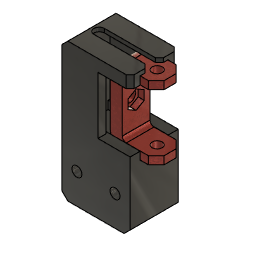
A Belt Tension Buddy_1x (Autodesk Fusion 360 design; units mm, degrees)
Autodesk Fusion 360 part; units mm, degrees
sketch "Sketch1" plane through (0, 0, 0) normal (0, 1, 0) x (1, 0, 0)
  line L0 (-15, 17.25) -> (15, 17.25)
  line L1 (15, 17.25) -> (15, -17.25)
  line L2 (15, -17.25) -> (-15, -17.25)
  line L3 (-15, -17.25) -> (-15, 17.25)
  line L4 (-15, 17.25) -> (15, -17.25) construction
  line L5 (15, 17.25) -> (-15, -17.25) construction
  line L6 (15, -17.25) -> (-15, -17.25)
  line L7 (-15, -17.25) -> (-15, -21.75)
  line L8 (-15, -21.75) -> (15, -21.75)
  line L9 (15, -21.75) -> (15, -17.25)
  dimension "d5316" = 30
  dimension "d5317" = 34.5
  dimension "d5318" = 4.5
  constraint horizontal L0
  constraint perpendicular L0 L1
  constraint parallel L0 L2
  constraint parallel L1 L3
  constraint coincident L4 origin
  constraint coincident L5 origin
  constraint horizontal L6
  constraint vertical L7
  constraint horizontal L8
  constraint vertical L9
  constraint coincident L2.end L3.start
  measures "d5316" distance of L1.end L2.end
  measures "d5317" distance of L0.end L1.end
  measures "d5318" distance of L1.end L8.end
extrude "Extrude1" add sketch "Sketch1" along normal mid plane 24 contours L0 L1 L2 L3 L6 makes body 1
sketch "Sketch15" plane through (-15, 0, 0) normal (-1, 0, 0) x (0, -1, 0)
  line L0 (12, -17.25) -> (12, 17.25)
  line L1 (-12, 17.25) -> (-12, -17.25)
  line L2 (-12, -17.25) -> (12, -17.25)
  line L3 (-12, 17.25) -> (12, 17.25)
  line L4 (12, 17.25) -> (12, 45.75)
  line L5 (12, 45.75) -> (-12, 45.75)
  line L6 (-12, 45.75) -> (-12, 17.25)
  line L7 (-12, 45.75) -> (12, 45.75)
  line L8 (12, 45.75) -> (12, 49.75)
  line L9 (12, 49.75) -> (-12, 49.75)
  line L10 (-12, 49.75) -> (-12, 45.75)
  line L11 (12, 17.25) -> (-12, 17.25)
  dimension "d5606" = 28.5
  dimension "d5609" = 4
  constraint horizontal L3
  constraint vertical L4
  constraint horizontal L5
  constraint vertical L6
  constraint coincident L1.start L3.start
  constraint coincident L0 L3.end
  constraint horizontal L7
  constraint vertical L8
  constraint horizontal L9
  constraint vertical L10
  constraint coincident L4.end L5.start
  measures "d5606" distance of L1.start L5.end
  measures "d5609" distance of L5.end L9.end
extrude "Extrude14" add sketch "Sketch15" along normal blind 4 contours L0 L1 L2 L3 L11 | L3 L4 L5 L6 L7 L11 bodies 1
extrude "Extrude15" add sketch "Sketch15" along normal blind 4 and the other way up to surface (30 mm away) contours L5 L7 L8 L9 L10 bodies 1
sketch "Sketch16" plane through (0, -12, 0) normal (0, -1, 0) x (1, 0, 0)
  line L0 (15, -17.25) -> (15, 17.25)
  line L1 (15, 17.25) -> (-15, 17.25)
  line L2 (-15, 17.25) -> (-15, 45.75)
  line L3 (-15, 45.75) -> (15, 45.75)
  line L4 (15, 45.75) -> (15, 49.75)
  line L5 (15, 49.75) -> (-19, 49.75)
  line L6 (-19, 49.75) -> (-19, -17.25)
  line L7 (-19, -17.25) -> (15, -17.25)
  line L8 (-19, 49.75) -> (15, 49.75)
  line L9 (15, 49.75) -> (15, -17.25)
  line L10 (15, -17.25) -> (-19, -17.25)
  line L11 (-19, -17.25) -> (-19, 49.75)
  constraint horizontal L8
  constraint vertical L9
  constraint horizontal L10
  constraint vertical L11
  constraint coincident L0.start L7.end
  constraint coincident L5.end L6.start
extrude "Extrude16" add sketch "Sketch16" against normal blind 4 contours L1 L2 L3 L9 bodies 1
mirror "Mirror2" about plane through (0, 0, 0) normal (0, 1, 0) of "Extrude16"
sketch "Sketch17" plane through (-15, 0, 0) normal (1, 0, 0) x (0, 1, 0)
  line L0 (8, 17.25) -> (8, 45.75)
  line L1 (8, 45.75) -> (-8, 45.75)
  line L2 (-8, 45.75) -> (-8, 17.25)
  line L3 (-8, 17.25) -> (8, 17.25)
  line L4 (-12, 49.75) -> (12, 49.75)
  line L5 (12, 49.75) -> (12, -17.25)
  line L6 (12, -17.25) -> (-12, -17.25)
  line L7 (-12, -17.25) -> (-12, 49.75)
  line L8 (-7, 49.75) -> (7, 49.75)
  line L9 (7, 49.75) -> (7, 13.25)
  line L10 (7, 13.25) -> (-7, 13.25)
  line L11 (-7, 13.25) -> (-7, 49.75)
  line L12 (0, 45.75) -> (0, 17.25) construction
  dimension "d5618" = 14
  dimension "d5619" = 4
  constraint horizontal L8
  constraint vertical L9
  constraint horizontal L10
  constraint vertical L11
  constraint coincident L4 L8.start
  constraint midpoint L1 L12.start
  constraint midpoint L3 L12.end
  constraint symmetric L9 L11 L12
  measures "d5618" distance of L9.end L10.end
  measures "d5619" distance of L3 L10
extrude "Extrude17" cut sketch "Sketch17" along normal up to surface (30 mm away) contours L3 L9 L10 L11 | L1 L3 L9 L11 | L1 L4 L8 L9 L11 bodies 1
sketch "Sketch18" plane through (-15, 0, 0) normal (1, 0, 0) x (0, 1, 0)
  line L0 (8, 17.25) -> (8, 45.75)
  line L1 (7, 49.75) -> (-7, 49.75)
  line L2 (-7, 49.75) -> (-7, 45.75)
  line L3 (-7, 13.25) -> (7, 13.25)
  line L4 (-8, 31.5) -> (8, 31.5)
  circle A0 centre (0, 31.5) radius 2.5
  line L5 (7, 17.25) -> (8, 17.25)
  line L6 (8, 45.75) -> (7, 45.75)
  line L7 (7, 45.75) -> (7, 49.75)
  line L8 (-7, 45.75) -> (-8, 45.75)
  line L9 (-8, 45.75) -> (-8, 17.25)
  line L10 (-8, 17.25) -> (-7, 17.25)
  line L11 (-7, 17.25) -> (-7, 13.25)
  line L12 (7, 13.25) -> (7, 17.25)
  dimension "d5622" = 5
  constraint midpoint L0 L4.end
  constraint midpoint L4 A0.centre
  measures "d5622" diameter of A0
hole "Hole7" at (-15, 0, 31.5) direction (-1, 0, 0) diameter 5 depth 13 tip angle 118 bodies 1
sketch "Sketch19" plane through (0, 0, 49.75) normal (0, 0, 1) x (-1, 0, 0)
  line L0 (15, -7) -> (-15, -7)
  line L1 (-15, -7) -> (-15, -12)
  line L2 (-15, -12) -> (19, -12)
  line L3 (19, -12) -> (19, 12)
  line L4 (19, 12) -> (-15, 12)
  line L5 (-15, 12) -> (-15, 7)
  line L6 (-15, 7) -> (15, 7)
  line L7 (15, 7) -> (15, -7)
  line L8 (-15, -12) -> (-15, 12)
  line L9 (-15, -2.6) -> (12.4, -2.6)
  arc A0 (12.4, -2.6) -> (12.4, 2.6) centre (12.4, 0) ccw
  line L10 (12.4, 2.6) -> (-15, 2.6)
  arc A1 (-15, 2.6) -> (-15, -2.6) centre (-15, 0) ccw
  line L11 (-15, 0) -> (12.4, 0) construction
  dimension "d5626" = 5.2
  constraint coincident L1.end L2.start
  constraint coincident L4.end L5.start
  constraint tangent L9 A0
  constraint tangent A0 L10
  constraint parallel L9 L10
  constraint tangent L10 A1
  constraint tangent L9 A1
  constraint perpendicular L8 L11
  constraint midpoint L8 A1.centre
  constraint tangent L7 A0
  measures "d5626" diameter of A0
extrude "Extrude18" add sketch "Sketch19" along normal blind 2 contours L0 L1 L2 L3 L4 L5 L6 L7 L8 | L0 L7 L8 L9 A0 | L6 L7 L8 A0 L10 bodies 1
sketch "Sketch20" plane through (0, 12, 0) normal (0, 1, 0) x (-1, 0, 0)
  line L0 (-15, 51.75) -> (-15, -17.25)
  line L1 (-15, -17.25) -> (19, -17.25)
  line L2 (19, -17.25) -> (19, 51.75)
  line L3 (19, 51.75) -> (-15, 51.75)
  line L4 (-15, 12.75) -> (19, 12.75)
  line L5 (2, 12.75) -> (2, -2.25)
  line L6 (2, -2.25) -> (11.5, -2.25)
  circle A0 centre (11.5, -2.25) radius 2.5
  circle A1 centre (11.5, -2.25) radius 5.5
  circle A2 centre (-7.5, -2.25) radius 2.5
  dimension "d5629" = 30
  dimension "d5630" = 15
  dimension "d5631" = 5
  dimension "d5632" = 11
  dimension "d5633" = 2
  constraint coincident L0 L4.start
  constraint coincident L2 L4.end
  constraint perpendicular L2 L4
  constraint midpoint L4 L5.start
  constraint perpendicular L4 L5
  constraint perpendicular L2 L6
  constraint coincident L6.end A0.centre
  constraint concentric A0 A1
  constraint symmetric L5 A0 A2
  measures "d5629" distance of L1 L4
  measures "d5630" distance of L1 L6
  measures "d5631" diameter of A0
  measures "d5632" diameter of A1
  measures "d5633" distance of L2 A1
hole "Hole8" at (-11.5, 12, -2.25) at (7.5, 12, -2.25) direction (0, -1, 0) diameter 5 depth 34 tip angle 118 counterbore diameter 11 counterbore depth 19 bodies 1
sketch "Sketch10" plane through (0, -7, 0) normal (0, 1, 0) x (-1, 0, 0)
  circle A0 centre (-7.5, -2.25) radius 2.5
  circle A1 centre (11.5, -2.25) radius 2.5
chamfer "Chamfer9" distance 1 angle 45 2 edges at (-9.5111, 12, -7.3778) (9.4889, 12, -7.3778) on bodies 1
sketch "Sketch22" plane through (0, 0, 0) normal (0, 1, 0) x (1, 0, 0)
  line L0 (-15, -45.75) -> (-15, -17.25)
  line L1 (-15, -17.25) -> (15, -17.25)
  line L2 (15, -17.25) -> (15, -45.75)
  line L3 (15, -45.75) -> (-15, -45.75)
  line L4 (-1, -45.75) -> (-1, -17.25)
  dimension "d5642" = 16
  constraint coincident L3 L4.start
  constraint coincident L1 L4.end
  constraint perpendicular L1 L4
  measures "d5642" distance of L2 L4
extrude "Extrude20" cut sketch "Sketch22" along normal mid plane 46 contours L1 L2 L3 L4 bodies 1
chamfer "Chamfer10" distance 2 angle 45 4 edges at (15, -2.6, 50.75) (15, 2.6, 50.75) (15, 12, 48.75) (15, -12, 48.75) on bodies 1
chamfer "Chamfer10" distance 3 angle 45 3 edges at (15, 0, -17.25) (-19, 0, -17.25) (-19, 0, 51.75) on bodies 1
sketch "Sketch1 (2)" plane through (0, 0, 0) normal (1, 0, 0) x (0, 1, 0) in component "AB Tension Fork_2x"
  line L0 (-16, 46.5) -> (7, 46.5)
  line L1 (7, 46.5) -> (7, 10)
  line L2 (7, 10) -> (-16, 10)
  line L3 (-16, 10) -> (-16, 14)
  line L4 (-16, 14) -> (1, 14)
  line L5 (1, 14) -> (1, 42.5)
  line L6 (1, 42.5) -> (-16, 42.5)
  line L7 (-16, 42.5) -> (-16, 46.5)
  line L8 (0, 0) -> (0, 10)
  dimension "d5367" = 4
  dimension "d5368" = 28.5
  dimension "d5369" = 10
  dimension "d5370" = 16
  dimension "d5371" = 4
  dimension "d5372" = 17
  dimension "d5373" = 6
  constraint horizontal L0
  constraint perpendicular L0 L1
  constraint perpendicular L1 L2
  constraint perpendicular L2 L3
  constraint perpendicular L3 L4
  constraint perpendicular L4 L5
  constraint perpendicular L3 L6
  constraint perpendicular L0 L7
  constraint coincident L0.start L7.end
  constraint coincident L8.start origin
  constraint coincident L2 L8.end
  constraint perpendicular L2 L8
  constraint equal L4 L6
  measures "d5367" distance of L6.end L0.start
  measures "d5368" distance of L4.end L5.end
  measures "d5369" distance of L8.start L8.end
  measures "d5370" distance of L3 L8
  measures "d5371" distance of L2.end L3.end
  measures "d5372" distance of L3.end L4.end
  measures "d5373" distance of L1 L5
extrude "Extrude1'" add sketch "Sketch1 (2)" along normal mid plane 13.8 separate body makes body 2 in component "AB Tension Fork_2x"
sketch "Sketch4" plane through (0, 1, 0) normal (0, -1, 0) x (1, 0, 0) in component "AB Tension Fork_2x"
  line L0 (-6.9, 14) -> (6.9, 14)
  line L1 (6.9, 14) -> (6.9, 42.5)
  line L2 (6.9, 42.5) -> (-6.9, 42.5)
  line L3 (-6.9, 42.5) -> (-6.9, 14)
  line L4 (0, 42.5) -> (0, 14) construction
  circle A0 centre (0, 28.25) radius 2.5 construction
  line L5 (4, 25.9406) -> (4, 30.5594)
  line L6 (4, 30.5594) -> (0, 32.8688)
  line L7 (0, 32.8688) -> (-4, 30.5594)
  line L8 (-4, 30.5594) -> (-4, 25.9406)
  line L9 (-4, 25.9406) -> (0, 23.6312)
  line L10 (0, 23.6312) -> (4, 25.9406)
  point P0 (0, 28.25)
  dimension "d5392" = 5
  dimension "d5470" = 4
  constraint midpoint L2 L4.start
  constraint midpoint L0 L4.end
  constraint midpoint L4 P0
  constraint coincident P0 A0.centre
  constraint vertical L5
  measures "d5392" diameter of A0
  measures "d5470" distance of P0 L10
hole "Hole1" at (0, 1, 28.25) direction (0, 1, 0) diameter 5.5 depth 16 tip angle 118 bodies 2 in component "AB Tension Fork_2x"
extrude "Extrude5" cut sketch "Sketch4" against normal blind 3 contours L5 L6 L7 L8 L9 L10 bodies 2 in component "AB Tension Fork_2x"
fillet "Fillet1" radius 2 2 edges at (0, 1, 42.5) (0, 1, 14) on bodies 2 in component "AB Tension Fork_2x"
fillet "Fillet1" radius 6 2 edges at (0, 7, 10) (0, 7, 46.5) on bodies 2 in component "AB Tension Fork_2x"
chamfer "Chamfer1" distance 4 angle 45 4 edges at (-6.9, -16, 44.5) (6.9, -16, 44.5) (-6.9, -16, 12) (6.9, -16, 12) on bodies 2 in component "AB Tension Fork_2x"
sketch "Sketch3" plane through (0, 0, 46.5) normal (0, 0, 1) x (-1, 0, 0) in component "AB Tension Fork_2x"
  line L0 (-2.9, 16) -> (-6.9, 12)
  line L1 (-6.9, 12) -> (-6.9, -1)
  line L2 (-6.9, -1) -> (6.9, -1)
  line L3 (6.9, -1) -> (6.9, 12)
  line L4 (6.9, 12) -> (2.9, 16)
  line L5 (2.9, 16) -> (-2.9, 16)
  line L6 (-2.9, 16) -> (-6.9, 12)
  line L7 (2.9, 16) -> (-2.9, 16)
  line L8 (6.9, 12) -> (2.9, 16)
  line L9 (6.9, -1) -> (6.9, 12)
  line L10 (-6.9, 12) -> (-6.9, -1)
  line L11 (6.9, -1) -> (6.9, -7)
  line L12 (6.9, -7) -> (-6.9, -7)
  line L13 (-6.9, -7) -> (-6.9, -1)
  line L14 (0, 0) -> (0, 9.5) construction
  circle A0 centre (0, 9.5) radius 2.5
  dimension "d5383" = 5
  dimension "d5384" = 4
  dimension "d5385" = 4.4
  constraint coincident L14.start origin
  constraint parallel L10 L14
  constraint coincident L14.end A0.centre
  measures "d5383" diameter of A0
  measures "d5384" distance of L7 A0
  measures "d5385" distance of L1 A0
extrude "Extrude3" cut sketch "Sketch3" against normal up to surface (36.5 mm away) contours A0 bodies 2 in component "AB Tension Fork_2x"
move_face "OffsetFaces1" offset -0.1 4 faces at (0.0623, -1.669, 46.5) (-0.0623, -1.669, 10) (-0.9667, -16, 43.8333) (-0.9667, -16, 11.3333) on bodies 2 in component "AB Tension Fork_2x"
cylinder "CylinderPrimitive1" add diameter 8 height 12.5 placed x (1, 0, 0) y (0, 1, 0) z (0, 0, 1) at (0, 0, 0) separate body makes body 3 in component "Idler Spacer"
hole "Hole1'" at (0, 0, 12.5) direction (0, 0, -1) diameter 5 depth 17 tip angle 180 bodies 3 in component "Idler Spacer"
component "AB Tension Fork_2x" placed x (0, 1, 0) y (-1, 0, 0) z (0, 0, 1) at (7, 0, 3.25)
component "Idler Spacer" placed x (0, -1, 0) y (1, 0, 0) z (0, 0, 1) at (0, 7, -3.25) in component "AB Tension Fork_2x"
equation "d5317 = frameProfile_1 + 4.5 mm + 10 mm"
equation "d5367 = Part_Thickness"
equation "d5368 = 2 * idler_height_gates + 2 * idler_shim_thickness - idler_gates_flange_thickness"
equation "d5371 = Part_Thickness"
equation "d5384 = Part_Thickness"
equation "d5606 = 2 * idler_height_gates + 2 * idler_shim_thickness - idler_gates_flange_thickness"
equation "d5607 = Part_Thickness"
equation "d5609 = Part_Thickness"
equation "d5610 = Part_Thickness"
equation "d5614 = -Part_Thickness"
equation "d5619 = Part_Thickness"
equation "frameProfile_1 = 20 mm"
equation "Part_Thickness = 4 mm" comment "Thickness of Printed Parts"
equation "idler_height_gates = 14 mm" comment "Gates 2GT Idler Height"
equation "idler_shim_thickness = 1 mm" comment "Shim Idler Thickness"
equation "idler_gates_flange_thickness = 1.5 mm" comment "Gates Idler Pulley Flange Thickness"
